Autodesk Inventor part; units mm, degrees
(part 3 of 3)
sketch "Sketch5" plane through (203.2, 0, 0) normal (0, 0, -1) x (-1, 0, 0)
  line L0 (0, 0) -> (203.2, 0) projected
  line L1 (0, 0) -> (0, -25.4) projected
  line L2 (203.2, -25.4) -> (0, -25.4) projected
  line L3 (203.2, 0) -> (203.2, -25.4) projected
  line L4 (12.7, -4.254) -> (190.5, -4.254) construction
  line L5 (190.5, -4.254) -> (190.5, -21.146) construction
  line L6 (190.5, -21.146) -> (12.7, -21.146) construction
  line L7 (12.7, -21.146) -> (12.7, -4.254) construction
  line L8 (18.2258, -17.272) -> (18.2258, -9.2099)
  line L9 (18.2258, -9.2099) -> (15.1581, -9.2099)
  line L10 (15.1581, -9.2099) -> (15.1581, -8.128)
  line L11 (15.1581, -8.128) -> (22.5088, -8.128)
  line L12 (22.5088, -8.128) -> (22.5088, -9.2099)
  line L13 (22.5088, -9.2099) -> (19.4411, -9.2099)
  line L14 (19.4411, -9.2099) -> (19.4411, -17.272)
  line L15 (19.4411, -17.272) -> (18.2258, -17.272)
  line L16 (30.5117, -17.272) -> (28.9334, -17.272)
  line L17 (28.9334, -17.272) -> (26.0434, -13.6337)
  line L18 (26.0434, -13.6337) -> (24.6504, -13.6337)
  line L19 (24.6504, -13.6337) -> (24.6504, -17.272)
  line L20 (24.6504, -17.272) -> (23.4351, -17.272)
  line L21 (23.4351, -17.272) -> (23.4351, -8.128)
  line L22 (23.4351, -8.128) -> (25.7915, -8.128)
  spline S0 degree 2 poles (25.7915, -8.128) (26.577, -8.128) (27.6366, -8.2984) (28.1183, -8.6097) knots 0 0 0 1 2 2 2
  spline S1 degree 2 poles (28.1183, -8.6097) (28.5999, -8.9209) (29.1557, -9.8916) (29.1557, -10.6104) knots 0 0 0 1 2 2 2
  spline S2 degree 2 poles (29.1557, -10.6104) (29.1557, -11.6107) (28.1331, -12.9668) (27.2587, -13.2928) knots 0 0 0 1 2 2 2
  line L23 (27.2587, -13.2928) -> (30.5117, -17.272)
  spline S3 degree 2 poles (27.8885, -10.7067) (27.8885, -10.3066) (27.607, -9.6915) (27.3106, -9.4914) knots 0 0 0 1 2 2 2
  spline S4 degree 2 poles (27.3106, -9.4914) (27.0512, -9.321) (26.3621, -9.1802) (25.8582, -9.1802) knots 0 0 0 1 2 2 2
  line L24 (25.8582, -9.1802) -> (24.6504, -9.1802)
  line L25 (24.6504, -9.1802) -> (24.6504, -12.6185)
  line L26 (24.6504, -12.6185) -> (25.7174, -12.6185)
  spline S5 degree 2 poles (25.7174, -12.6185) (26.2435, -12.6185) (27.0808, -12.4332) (27.3698, -12.1442) knots 0 0 0 1 2 2 2
  spline S6 degree 2 poles (27.3698, -12.1442) (27.6366, -11.8923) (27.8885, -11.1809) (27.8885, -10.7067) knots 0 0 0 1 2 2 2
  line L27 (31.2379, -17.272) -> (31.2379, -8.128)
  line L28 (31.2379, -8.128) -> (36.9584, -8.128)
  line L29 (36.9584, -8.128) -> (36.9584, -9.2099)
  line L30 (36.9584, -9.2099) -> (32.4531, -9.2099)
  line L31 (32.4531, -9.2099) -> (32.4531, -11.7145)
  line L32 (32.4531, -11.7145) -> (36.6546, -11.7145)
  line L33 (36.6546, -11.7145) -> (36.6546, -12.7963)
  line L34 (36.6546, -12.7963) -> (32.4531, -12.7963)
  line L35 (32.4531, -12.7963) -> (32.4531, -16.1901)
  line L36 (32.4531, -16.1901) -> (36.9584, -16.1901)
  line L37 (36.9584, -16.1901) -> (36.9584, -17.272)
  line L38 (36.9584, -17.272) -> (31.2379, -17.272)
  spline S7 degree 2 poles (44.4945, -14.4636) (44.4945, -15.1453) (43.9758, -16.1901) (43.546, -16.531) knots 0 0 0 1 2 2 2
  spline S8 degree 2 poles (43.546, -16.531) (43.0273, -16.9311) (41.8491, -17.272) (40.9154, -17.272) knots 0 0 0 1 2 2 2
  line L39 (40.9154, -17.272) -> (38.2923, -17.272)
  line L40 (38.2923, -17.272) -> (38.2923, -8.128)
  line L41 (38.2923, -8.128) -> (40.7153, -8.128)
  spline S9 degree 2 poles (40.7153, -8.128) (41.6935, -8.128) (42.6716, -8.254) (43.1162, -8.4985) knots 0 0 0 1 2 2 2
  spline S10 degree 2 poles (43.1162, -8.4985) (43.6127, -8.7579) (44.0647, -9.61) (44.0647, -10.188) knots 0 0 0 1 2 2 2
  spline S11 degree 2 poles (44.0647, -10.188) (44.0647, -10.8327) (43.383, -11.8553) (42.7827, -12.1442) knots 0 0 0 1 2 2 2
  line L42 (42.7827, -12.1442) -> (42.7827, -12.1887)
  spline S12 degree 2 poles (42.7827, -12.1887) (43.5978, -12.411) (44.4945, -13.5892) (44.4945, -14.4636) knots 0 0 0 1 2 2 2
  spline S13 degree 2 poles (43.2273, -14.5155) (43.2273, -13.9968) (42.9309, -13.3299) (42.4863, -13.0927) knots 0 0 0 1 2 2 2
  spline S14 degree 2 poles (42.4863, -13.0927) (42.1973, -12.9445) (41.5156, -12.8556) (40.8858, -12.8556) knots 0 0 0 1 2 2 2
  line L43 (40.8858, -12.8556) -> (39.5075, -12.8556)
  line L44 (39.5075, -12.8556) -> (39.5075, -16.2346)
  line L45 (39.5075, -16.2346) -> (40.493, -16.2346)
  spline S15 degree 2 poles (40.493, -16.2346) (41.2933, -16.2346) (42.2122, -16.0864) (42.5679, -15.8493) knots 0 0 0 1 2 2 2
  spline S16 degree 2 poles (42.5679, -15.8493) (42.9087, -15.6047) (43.2273, -14.9971) (43.2273, -14.5155) knots 0 0 0 1 2 2 2
  spline S17 degree 2 poles (42.7976, -10.3584) (42.7976, -10.0324) (42.5753, -9.5433) (42.3307, -9.4025) knots 0 0 0 1 2 2 2
  spline S18 degree 2 poles (42.3307, -9.4025) (42.0343, -9.2395) (41.3156, -9.1654) (40.6709, -9.1654) knots 0 0 0 1 2 2 2
  line L46 (40.6709, -9.1654) -> (39.5075, -9.1654)
  line L47 (39.5075, -9.1654) -> (39.5075, -11.8404)
  line L48 (39.5075, -11.8404) -> (40.8858, -11.8404)
  spline S19 degree 2 poles (40.8858, -11.8404) (41.4563, -11.8404) (41.9973, -11.7219) (42.2863, -11.5366) knots 0 0 0 1 2 2 2
  spline S20 degree 2 poles (42.2863, -11.5366) (42.5679, -11.3588) (42.7976, -10.7882) (42.7976, -10.3584) knots 0 0 0 1 2 2 2
  line L49 (51.0005, -17.272) -> (45.7023, -17.272)
  line L50 (45.7023, -17.272) -> (45.7023, -8.128)
  line L51 (45.7023, -8.128) -> (46.9175, -8.128)
  line L52 (46.9175, -8.128) -> (46.9175, -16.1901)
  line L53 (46.9175, -16.1901) -> (51.0005, -16.1901)
  line L54 (51.0005, -16.1901) -> (51.0005, -17.272)
  line L55 (51.9564, -17.272) -> (51.9564, -8.128)
  line L56 (51.9564, -8.128) -> (57.6769, -8.128)
  line L57 (57.6769, -8.128) -> (57.6769, -9.2099)
  line L58 (57.6769, -9.2099) -> (53.1716, -9.2099)
  line L59 (53.1716, -9.2099) -> (53.1716, -11.7145)
  line L60 (53.1716, -11.7145) -> (57.3731, -11.7145)
  line L61 (57.3731, -11.7145) -> (57.3731, -12.7963)
  line L62 (57.3731, -12.7963) -> (53.1716, -12.7963)
  line L63 (53.1716, -12.7963) -> (53.1716, -16.1901)
  line L64 (53.1716, -16.1901) -> (57.6769, -16.1901)
  line L65 (57.6769, -16.1901) -> (57.6769, -17.272)
  line L66 (57.6769, -17.272) -> (51.9564, -17.272)
  line L67 (68.4067, -9.2099) -> (64.1533, -9.2099)
  line L68 (64.1533, -9.2099) -> (64.1533, -11.7886)
  line L69 (64.1533, -11.7886) -> (68.2288, -11.7886)
  line L70 (68.2288, -11.7886) -> (68.2288, -12.8704)
  line L71 (68.2288, -12.8704) -> (64.1533, -12.8704)
  line L72 (64.1533, -12.8704) -> (64.1533, -17.272)
  line L73 (64.1533, -17.272) -> (62.9381, -17.272)
  line L74 (62.9381, -17.272) -> (62.9381, -8.128)
  line L75 (62.9381, -8.128) -> (68.4067, -8.128)
  line L76 (68.4067, -8.128) -> (68.4067, -9.2099)
  spline S21 degree 2 poles (75.9649, -9.1728) (76.4836, -9.7804) (77.0616, -11.5589) (77.0616, -12.7) knots 0 0 0 1 2 2 2
  spline S22 degree 2 poles (77.0616, -12.7) (77.0616, -13.8115) (76.4985, -15.6121) (75.9649, -16.2198) knots 0 0 0 1 2 2 2
  spline S23 degree 2 poles (75.9649, -16.2198) (75.4018, -16.857) (73.9124, -17.4647) (73.0157, -17.4647) knots 0 0 0 1 2 2 2
  spline S24 degree 2 poles (73.0157, -17.4647) (72.0895, -17.4647) (70.6075, -16.8348) (70.0665, -16.2198) knots 0 0 0 1 2 2 2
  spline S25 degree 2 poles (70.0665, -16.2198) (69.5404, -15.6121) (68.9773, -13.8263) (68.9773, -12.7) knots 0 0 0 1 2 2 2
  spline S26 degree 2 poles (68.9773, -12.7) (68.9773, -11.5514) (69.5478, -9.8027) (70.074, -9.1728) knots 0 0 0 1 2 2 2
  spline S27 degree 2 poles (70.074, -9.1728) (70.6075, -8.5652) (72.0969, -7.9353) (73.0157, -7.9353) knots 0 0 0 1 2 2 2
  spline S28 degree 2 poles (73.0157, -7.9353) (73.9494, -7.9353) (75.4462, -8.5874) (75.9649, -9.1728) knots 0 0 0 1 2 2 2
  spline S29 degree 2 poles (75.7945, -12.7) (75.7945, -11.796) (75.4018, -10.3955) (75.0461, -9.9361) knots 0 0 0 1 2 2 2
  spline S30 degree 2 poles (75.0461, -9.9361) (74.683, -9.4618) (73.6604, -8.9876) (73.0231, -8.9876) knots 0 0 0 1 2 2 2
  spline S31 degree 2 poles (73.0231, -8.9876) (72.3637, -8.9876) (71.3707, -9.447) (70.9928, -9.9361) knots 0 0 0 1 2 2 2
  spline S32 degree 2 poles (70.9928, -9.9361) (70.6297, -10.4029) (70.2444, -11.8108) (70.2444, -12.7) knots 0 0 0 1 2 2 2
  spline S33 degree 2 poles (70.2444, -12.7) (70.2444, -14.5006) (71.756, -16.4124) (73.0231, -16.4124) knots 0 0 0 1 2 2 2
  spline S34 degree 2 poles (73.0231, -16.4124) (74.2903, -16.4124) (75.7945, -14.5006) (75.7945, -12.7) knots 0 0 0 1 2 2 2
  spline S35 degree 2 poles (81.5892, -17.4647) (80.7815, -17.4647) (79.581, -17.0423) (79.1587, -16.6199) knots 0 0 0 1 2 2 2
  spline S36 degree 2 poles (79.1587, -16.6199) (78.677, -16.1457) (78.2843, -14.8119) (78.2843, -13.8337) knots 0 0 0 1 2 2 2
  line L77 (78.2843, -13.8337) -> (78.2843, -8.128)
  line L78 (78.2843, -8.128) -> (79.4995, -8.128)
  line L79 (79.4995, -8.128) -> (79.4995, -13.8337)
  spline S37 degree 2 poles (79.4995, -13.8337) (79.4995, -14.471) (79.6626, -15.3306) (79.8923, -15.6788) knots 0 0 0 1 2 2 2
  spline S38 degree 2 poles (79.8923, -15.6788) (80.1368, -16.0493) (80.9815, -16.4273) (81.5892, -16.4273) knots 0 0 0 1 2 2 2
  spline S39 degree 2 poles (81.5892, -16.4273) (82.1597, -16.4273) (83.0489, -16.0493) (83.2935, -15.6788) knots 0 0 0 1 2 2 2
  spline S40 degree 2 poles (83.2935, -15.6788) (83.5232, -15.3306) (83.6862, -14.4784) (83.6862, -13.8634) knots 0 0 0 1 2 2 2
  line L80 (83.6862, -13.8634) -> (83.6862, -8.128)
  line L81 (83.6862, -8.128) -> (84.9015, -8.128)
  line L82 (84.9015, -8.128) -> (84.9015, -13.8337)
  spline S41 degree 2 poles (84.9015, -13.8337) (84.9015, -14.7896) (84.5161, -16.1531) (84.0271, -16.6199) knots 0 0 0 1 2 2 2
  spline S42 degree 2 poles (84.0271, -16.6199) (83.5899, -17.0497) (82.4339, -17.4647) (81.5892, -17.4647) knots 0 0 0 1 2 2 2
  line L83 (93.7194, -17.272) -> (92.1411, -17.272)
  line L84 (92.1411, -17.272) -> (89.2512, -13.6337)
  line L85 (89.2512, -13.6337) -> (87.8581, -13.6337)
  line L86 (87.8581, -13.6337) -> (87.8581, -17.272)
  line L87 (87.8581, -17.272) -> (86.6428, -17.272)
  line L88 (86.6428, -17.272) -> (86.6428, -8.128)
  line L89 (86.6428, -8.128) -> (88.9992, -8.128)
  spline S43 degree 2 poles (88.9992, -8.128) (89.7847, -8.128) (90.8443, -8.2984) (91.326, -8.6097) knots 0 0 0 1 2 2 2
  spline S44 degree 2 poles (91.326, -8.6097) (91.8076, -8.9209) (92.3634, -9.8916) (92.3634, -10.6104) knots 0 0 0 1 2 2 2
  spline S45 degree 2 poles (92.3634, -10.6104) (92.3634, -11.6107) (91.3408, -12.9668) (90.4664, -13.2928) knots 0 0 0 1 2 2 2
  line L90 (90.4664, -13.2928) -> (93.7194, -17.272)
  spline S46 degree 2 poles (91.0963, -10.7067) (91.0963, -10.3066) (90.8147, -9.6915) (90.5183, -9.4914) knots 0 0 0 1 2 2 2
  spline S47 degree 2 poles (90.5183, -9.4914) (90.2589, -9.321) (89.5698, -9.1802) (89.0659, -9.1802) knots 0 0 0 1 2 2 2
  line L91 (89.0659, -9.1802) -> (87.8581, -9.1802)
  line L92 (87.8581, -9.1802) -> (87.8581, -12.6185)
  line L93 (87.8581, -12.6185) -> (88.9251, -12.6185)
  spline S48 degree 2 poles (88.9251, -12.6185) (89.4512, -12.6185) (90.2886, -12.4332) (90.5776, -12.1442) knots 0 0 0 1 2 2 2
  spline S49 degree 2 poles (90.5776, -12.1442) (90.8443, -11.8923) (91.0963, -11.1809) (91.0963, -10.7067) knots 0 0 0 1 2 2 2
  line L94 (97.6319, -17.272) -> (94.0899, -17.272)
  line L95 (94.0899, -17.272) -> (94.0899, -16.3383)
  line L96 (94.0899, -16.3383) -> (95.2533, -16.3383)
  line L97 (95.2533, -16.3383) -> (95.2533, -9.0617)
  line L98 (95.2533, -9.0617) -> (94.0899, -9.0617)
  line L99 (94.0899, -9.0617) -> (94.0899, -8.128)
  line L100 (94.0899, -8.128) -> (97.6319, -8.128)
  line L101 (97.6319, -8.128) -> (97.6319, -9.0617)
  line L102 (97.6319, -9.0617) -> (96.4685, -9.0617)
  line L103 (96.4685, -9.0617) -> (96.4685, -16.3383)
  line L104 (96.4685, -16.3383) -> (97.6319, -16.3383)
  line L105 (97.6319, -16.3383) -> (97.6319, -17.272)
  line L106 (99.1362, -17.272) -> (99.1362, -8.128)
  line L107 (99.1362, -8.128) -> (104.8567, -8.128)
  line L108 (104.8567, -8.128) -> (104.8567, -9.2099)
  line L109 (104.8567, -9.2099) -> (100.3514, -9.2099)
  line L110 (100.3514, -9.2099) -> (100.3514, -11.7145)
  line L111 (100.3514, -11.7145) -> (104.5529, -11.7145)
  line L112 (104.5529, -11.7145) -> (104.5529, -12.7963)
  line L113 (104.5529, -12.7963) -> (100.3514, -12.7963)
  line L114 (100.3514, -12.7963) -> (100.3514, -16.1901)
  line L115 (100.3514, -16.1901) -> (104.8567, -16.1901)
  line L116 (104.8567, -16.1901) -> (104.8567, -17.272)
  line L117 (104.8567, -17.272) -> (99.1362, -17.272)
  line L118 (113.2671, -17.272) -> (111.6888, -17.272)
  line L119 (111.6888, -17.272) -> (108.7989, -13.6337)
  line L120 (108.7989, -13.6337) -> (107.4058, -13.6337)
  line L121 (107.4058, -13.6337) -> (107.4058, -17.272)
  line L122 (107.4058, -17.272) -> (106.1905, -17.272)
  line L123 (106.1905, -17.272) -> (106.1905, -8.128)
  line L124 (106.1905, -8.128) -> (108.5469, -8.128)
  spline S50 degree 2 poles (108.5469, -8.128) (109.3324, -8.128) (110.392, -8.2984) (110.8737, -8.6097) knots 0 0 0 1 2 2 2
  spline S51 degree 2 poles (110.8737, -8.6097) (111.3553, -8.9209) (111.9111, -9.8916) (111.9111, -10.6104) knots 0 0 0 1 2 2 2
  spline S52 degree 2 poles (111.9111, -10.6104) (111.9111, -11.6107) (110.8885, -12.9668) (110.0141, -13.2928) knots 0 0 0 1 2 2 2
  line L125 (110.0141, -13.2928) -> (113.2671, -17.272)
  spline S53 degree 2 poles (110.644, -10.7067) (110.644, -10.3066) (110.3624, -9.6915) (110.066, -9.4914) knots 0 0 0 1 2 2 2
  spline S54 degree 2 poles (110.066, -9.4914) (109.8066, -9.321) (109.1175, -9.1802) (108.6136, -9.1802) knots 0 0 0 1 2 2 2
  line L126 (108.6136, -9.1802) -> (107.4058, -9.1802)
  line L127 (107.4058, -9.1802) -> (107.4058, -12.6185)
  line L128 (107.4058, -12.6185) -> (108.4728, -12.6185)
  spline S55 degree 2 poles (108.4728, -12.6185) (108.9989, -12.6185) (109.8363, -12.4332) (110.1253, -12.1442) knots 0 0 0 1 2 2 2
  spline S56 degree 2 poles (110.1253, -12.1442) (110.392, -11.8923) (110.644, -11.1809) (110.644, -10.7067) knots 0 0 0 1 2 2 2
  line L129 (120.0547, -17.272) -> (120.0547, -9.2099)
  line L130 (120.0547, -9.2099) -> (116.987, -9.2099)
  line L131 (116.987, -9.2099) -> (116.987, -8.128)
  line L132 (116.987, -8.128) -> (124.3377, -8.128)
  line L133 (124.3377, -8.128) -> (124.3377, -9.2099)
  line L134 (124.3377, -9.2099) -> (121.27, -9.2099)
  line L135 (121.27, -9.2099) -> (121.27, -17.272)
  line L136 (121.27, -17.272) -> (120.0547, -17.272)
  line L137 (132.3406, -17.272) -> (130.7622, -17.272)
  line L138 (130.7622, -17.272) -> (127.8723, -13.6337)
  line L139 (127.8723, -13.6337) -> (126.4792, -13.6337)
  line L140 (126.4792, -13.6337) -> (126.4792, -17.272)
  line L141 (126.4792, -17.272) -> (125.264, -17.272)
  line L142 (125.264, -17.272) -> (125.264, -8.128)
  line L143 (125.264, -8.128) -> (127.6204, -8.128)
  spline S57 degree 2 poles (127.6204, -8.128) (128.4059, -8.128) (129.4655, -8.2984) (129.9471, -8.6097) knots 0 0 0 1 2 2 2
  spline S58 degree 2 poles (129.9471, -8.6097) (130.4288, -8.9209) (130.9845, -9.8916) (130.9845, -10.6104) knots 0 0 0 1 2 2 2
  spline S59 degree 2 poles (130.9845, -10.6104) (130.9845, -11.6107) (129.962, -12.9668) (129.0876, -13.2928) knots 0 0 0 1 2 2 2
  line L144 (129.0876, -13.2928) -> (132.3406, -17.272)
  spline S60 degree 2 poles (129.7174, -10.7067) (129.7174, -10.3066) (129.4358, -9.6915) (129.1394, -9.4914) knots 0 0 0 1 2 2 2
  spline S61 degree 2 poles (129.1394, -9.4914) (128.8801, -9.321) (128.191, -9.1802) (127.6871, -9.1802) knots 0 0 0 1 2 2 2
  line L145 (127.6871, -9.1802) -> (126.4792, -9.1802)
  line L146 (126.4792, -9.1802) -> (126.4792, -12.6185)
  line L147 (126.4792, -12.6185) -> (127.5463, -12.6185)
  spline S62 degree 2 poles (127.5463, -12.6185) (128.0724, -12.6185) (128.9097, -12.4332) (129.1987, -12.1442) knots 0 0 0 1 2 2 2
  spline S63 degree 2 poles (129.1987, -12.1442) (129.4655, -11.8923) (129.7174, -11.1809) (129.7174, -10.7067) knots 0 0 0 1 2 2 2
  line L148 (132.0812, -17.272) -> (135.1638, -8.128)
  line L149 (135.1638, -8.128) -> (136.6606, -8.128)
  line L150 (136.6606, -8.128) -> (139.7432, -17.272)
  line L151 (139.7432, -17.272) -> (138.4613, -17.272)
  line L152 (138.4613, -17.272) -> (137.6314, -14.7155)
  line L153 (137.6314, -14.7155) -> (134.1412, -14.7155)
  line L154 (134.1412, -14.7155) -> (133.3113, -17.272)
  line L155 (133.3113, -17.272) -> (132.0812, -17.272)
  line L156 (137.2979, -13.6781) -> (135.8826, -9.3729)
  line L157 (135.8826, -9.3729) -> (134.4747, -13.6781)
  line L158 (134.4747, -13.6781) -> (137.2979, -13.6781)
  line L159 (147.1533, -17.272) -> (145.7898, -17.272)
  line L160 (145.7898, -17.272) -> (141.7439, -9.3877)
  line L161 (141.7439, -9.3877) -> (141.7439, -17.272)
  line L162 (141.7439, -17.272) -> (140.6102, -17.272)
  line L163 (140.6102, -17.272) -> (140.6102, -8.128)
  line L164 (140.6102, -8.128) -> (142.3367, -8.128)
  line L165 (142.3367, -8.128) -> (146.0195, -15.3676)
  line L166 (146.0195, -15.3676) -> (146.0195, -8.128)
  line L167 (146.0195, -8.128) -> (147.1533, -8.128)
  line L168 (147.1533, -8.128) -> (147.1533, -17.272)
  spline S64 degree 2 poles (151.5548, -17.435) (150.5619, -17.435) (149.1688, -17.0201) (148.5538, -16.7237) knots 0 0 0 1 2 2 2
  line L169 (148.5538, -16.7237) -> (148.5538, -15.1972)
  line L170 (148.5538, -15.1972) -> (148.6427, -15.1972)
  spline S65 degree 2 poles (148.6427, -15.1972) (149.2429, -15.7604) (150.762, -16.3828) (151.4659, -16.3828) knots 0 0 0 1 2 2 2
  spline S66 degree 2 poles (151.4659, -16.3828) (152.4737, -16.3828) (153.5037, -15.5455) (153.5037, -14.8563) knots 0 0 0 1 2 2 2
  spline S67 degree 2 poles (153.5037, -14.8563) (153.5037, -14.308) (152.9628, -13.6263) (152.3774, -13.4558) knots 0 0 0 1 2 2 2
  spline S68 degree 2 poles (152.3774, -13.4558) (151.955, -13.3373) (151.251, -13.1742) (150.7249, -13.0409) knots 0 0 0 1 2 2 2
  spline S69 degree 2 poles (150.7249, -13.0409) (150.2507, -12.9149) (149.5023, -12.537) (149.2133, -12.2332) knots 0 0 0 1 2 2 2
  spline S70 degree 2 poles (149.2133, -12.2332) (148.9317, -11.9294) (148.6205, -11.1142) (148.6205, -10.5807) knots 0 0 0 1 2 2 2
  spline S71 degree 2 poles (148.6205, -10.5807) (148.6205, -9.4692) (150.3544, -7.965) (151.6956, -7.965) knots 0 0 0 1 2 2 2
  spline S72 degree 2 poles (151.6956, -7.965) (152.4663, -7.965) (153.8297, -8.2688) (154.4151, -8.5578) knots 0 0 0 1 2 2 2
  line L171 (154.4151, -8.5578) -> (154.4151, -10.0102)
  line L172 (154.4151, -10.0102) -> (154.3262, -10.0102)
  spline S73 degree 2 poles (154.3262, -10.0102) (153.889, -9.61) (152.5256, -9.0172) (151.7771, -9.0172) knots 0 0 0 1 2 2 2
  spline S74 degree 2 poles (151.7771, -9.0172) (150.9324, -9.0172) (149.8876, -9.8101) (149.8876, -10.4548) knots 0 0 0 1 2 2 2
  spline S75 degree 2 poles (149.8876, -10.4548) (149.8876, -11.0327) (150.5026, -11.7219) (151.0806, -11.8775) knots 0 0 0 1 2 2 2
  spline S76 degree 2 poles (151.0806, -11.8775) (151.4659, -11.9812) (152.5848, -12.248) (152.9553, -12.3591) knots 0 0 0 1 2 2 2
  spline S77 degree 2 poles (152.9553, -12.3591) (153.8964, -12.6481) (154.7708, -13.8115) (154.7708, -14.6637) knots 0 0 0 1 2 2 2
  spline S78 degree 2 poles (154.7708, -14.6637) (154.7708, -15.2046) (154.3336, -16.242) (153.9409, -16.6051) knots 0 0 0 1 2 2 2
  spline S79 degree 2 poles (153.9409, -16.6051) (153.5037, -17.0052) (152.3922, -17.435) (151.5548, -17.435) knots 0 0 0 1 2 2 2
  line L173 (161.4769, -9.2099) -> (157.2235, -9.2099)
  line L174 (157.2235, -9.2099) -> (157.2235, -11.7886)
  line L175 (157.2235, -11.7886) -> (161.2991, -11.7886)
  line L176 (161.2991, -11.7886) -> (161.2991, -12.8704)
  line L177 (161.2991, -12.8704) -> (157.2235, -12.8704)
  line L178 (157.2235, -12.8704) -> (157.2235, -17.272)
  line L179 (157.2235, -17.272) -> (156.0083, -17.272)
  line L180 (156.0083, -17.272) -> (156.0083, -8.128)
  line L181 (156.0083, -8.128) -> (161.4769, -8.128)
  line L182 (161.4769, -8.128) -> (161.4769, -9.2099)
  spline S80 degree 2 poles (169.0351, -9.1728) (169.5539, -9.7804) (170.1318, -11.5589) (170.1318, -12.7) knots 0 0 0 1 2 2 2
  spline S81 degree 2 poles (170.1318, -12.7) (170.1318, -13.8115) (169.5687, -15.6121) (169.0351, -16.2198) knots 0 0 0 1 2 2 2
  spline S82 degree 2 poles (169.0351, -16.2198) (168.472, -16.857) (166.9826, -17.4647) (166.0859, -17.4647) knots 0 0 0 1 2 2 2
  spline S83 degree 2 poles (166.0859, -17.4647) (165.1597, -17.4647) (163.6777, -16.8348) (163.1367, -16.2198) knots 0 0 0 1 2 2 2
  spline S84 degree 2 poles (163.1367, -16.2198) (162.6106, -15.6121) (162.0475, -13.8263) (162.0475, -12.7) knots 0 0 0 1 2 2 2
  spline S85 degree 2 poles (162.0475, -12.7) (162.0475, -11.5514) (162.618, -9.8027) (163.1442, -9.1728) knots 0 0 0 1 2 2 2
  spline S86 degree 2 poles (163.1442, -9.1728) (163.6777, -8.5652) (165.1671, -7.9353) (166.0859, -7.9353) knots 0 0 0 1 2 2 2
  spline S87 degree 2 poles (166.0859, -7.9353) (167.0196, -7.9353) (168.5164, -8.5874) (169.0351, -9.1728) knots 0 0 0 1 2 2 2
  spline S88 degree 2 poles (168.8647, -12.7) (168.8647, -11.796) (168.472, -10.3955) (168.1163, -9.9361) knots 0 0 0 1 2 2 2
  spline S89 degree 2 poles (168.1163, -9.9361) (167.7532, -9.4618) (166.7306, -8.9876) (166.0934, -8.9876) knots 0 0 0 1 2 2 2
  spline S90 degree 2 poles (166.0934, -8.9876) (165.4339, -8.9876) (164.4409, -9.447) (164.063, -9.9361) knots 0 0 0 1 2 2 2
  spline S91 degree 2 poles (164.063, -9.9361) (163.6999, -10.4029) (163.3146, -11.8108) (163.3146, -12.7) knots 0 0 0 1 2 2 2
  spline S92 degree 2 poles (163.3146, -12.7) (163.3146, -14.5006) (164.8262, -16.4124) (166.0934, -16.4124) knots 0 0 0 1 2 2 2
  spline S93 degree 2 poles (166.0934, -16.4124) (167.3605, -16.4124) (168.8647, -14.5006) (168.8647, -12.7) knots 0 0 0 1 2 2 2
  line L183 (178.5422, -17.272) -> (176.9639, -17.272)
  line L184 (176.9639, -17.272) -> (174.074, -13.6337)
  line L185 (174.074, -13.6337) -> (172.6809, -13.6337)
  line L186 (172.6809, -13.6337) -> (172.6809, -17.272)
  line L187 (172.6809, -17.272) -> (171.4656, -17.272)
  line L188 (171.4656, -17.272) -> (171.4656, -8.128)
  line L189 (171.4656, -8.128) -> (173.822, -8.128)
  spline S94 degree 2 poles (173.822, -8.128) (174.6075, -8.128) (175.6671, -8.2984) (176.1488, -8.6097) knots 0 0 0 1 2 2 2
  spline S95 degree 2 poles (176.1488, -8.6097) (176.6304, -8.9209) (177.1862, -9.8916) (177.1862, -10.6104) knots 0 0 0 1 2 2 2
  spline S96 degree 2 poles (177.1862, -10.6104) (177.1862, -11.6107) (176.1636, -12.9668) (175.2892, -13.2928) knots 0 0 0 1 2 2 2
  line L190 (175.2892, -13.2928) -> (178.5422, -17.272)
  spline S97 degree 2 poles (175.9191, -10.7067) (175.9191, -10.3066) (175.6375, -9.6915) (175.3411, -9.4914) knots 0 0 0 1 2 2 2
  spline S98 degree 2 poles (175.3411, -9.4914) (175.0817, -9.321) (174.3926, -9.1802) (173.8887, -9.1802) knots 0 0 0 1 2 2 2
  line L191 (173.8887, -9.1802) -> (172.6809, -9.1802)
  line L192 (172.6809, -9.1802) -> (172.6809, -12.6185)
  line L193 (172.6809, -12.6185) -> (173.7479, -12.6185)
  spline S99 degree 2 poles (173.7479, -12.6185) (174.2741, -12.6185) (175.1114, -12.4332) (175.4004, -12.1442) knots 0 0 0 1 2 2 2
  spline S100 degree 2 poles (175.4004, -12.1442) (175.6671, -11.8923) (175.9191, -11.1809) (175.9191, -10.7067) knots 0 0 0 1 2 2 2
  line L194 (187.1083, -17.272) -> (185.893, -17.272)
  line L195 (185.893, -17.272) -> (185.893, -9.3951)
  line L196 (185.893, -9.3951) -> (183.507, -14.7526)
  line L197 (183.507, -14.7526) -> (182.766, -14.7526)
  line L198 (182.766, -14.7526) -> (180.4022, -9.3951)
  line L199 (180.4022, -9.3951) -> (180.4022, -17.272)
  line L200 (180.4022, -17.272) -> (179.2684, -17.272)
  line L201 (179.2684, -17.272) -> (179.2684, -8.128)
  line L202 (179.2684, -8.128) -> (180.9283, -8.128)
  line L203 (180.9283, -8.128) -> (183.2106, -13.2187)
  line L204 (183.2106, -13.2187) -> (185.4188, -8.128)
  line L205 (185.4188, -8.128) -> (187.1083, -8.128)
  line L206 (187.1083, -8.128) -> (187.1083, -17.272)
  dimension "d30" = 203.2
  dimension "d31" = 177.8
  dimension "d32" = 16.892
  dimension "d33" = 4.254
  dimension "d34" = 25.4
  dimension "d35" = 12.7
  constraints: 2 other
  measures "d30" distance of L0.start L0.end
  measures "d31" distance of L7.end L4.end
  measures "d32" distance of L7.start L7.end
  measures "d33" distance between parallel lines of L0 L4
  measures "d34" distance of L0.start L1.end
  measures "d35" distance between parallel lines of L1 L7
extrude "Extrusion5" cut sketch "Sketch5" against normal blind 5.08 contours L8 L9 L10 L11 L12 L13 L14 L15 | L16 L17 L18 L19 L20 L21 L22 S0 S1 S2 L23 | L27 L28 L29 L30 L31 L32 L33 L34 L35 L36 L37 L38 | S7 S8 L39 L40 L41 S9 S10 S11 L42 S12 | L49 L50 L51 L52 L53 L54 | L55 L56 L57 L58 L59 L60 L61 L62 L63 L64 L65 L66 | L67 L68 L69 L70 L71 L72 L73 L74 L75 L76 | S21 S22 S23 S24 S25 S26 S27 S28 | S35 S36 L77 L78 L79 S37 S38 S39 S40 L80 L81 L82 S41 S42 | L83 L84 L85 L86 L87 L88 L89 S43 S44 S45 L90 | L94 L95 L96 L97 L98 L99 L100 L101 L102 L103 L104 L105 | L106 L107 L108 L109 L110 L111 L112 L113 L114 L115 L116 L117 | L118 L119 L120 L121 L122 L123 L124 S50 S51 S52 L125 | L129 L130 L131 L132 L133 L134 L135 L136 | L137 L148 L144 | L144 L148 L149 L150 L151 L152 L153 L154 L155 | L137 L138 L139 L140 L141 L142 L143 S57 S58 S59 L144 L148 | L159 L160 L161 L162 L163 L164 L165 L166 L167 L168 | S64 L169 L170 S65 S66 S67 S68 S69 S70 S71 S72 L171 L172 S73 S74 S75 S76 S77 S78 S79 | L173 L174 L175 L176 L177 L178 L179 L180 L181 L182 | S80 S81 S82 S83 S84 S85 S86 S87 | L183 L184 L185 L186 L187 L188 L189 S94 S95 S96 L190 | L194 L195 L196 L197 L198 L199 L200 L201 L202 L203 L204 L205 L206
equation "\"d6\" = 0.5 * d3 - 0.5 * d5"
equation "\"d7\" = 0.5 * d2 - 0.5 * d4"
equation "\"d16\" = 0.5 * d15 - 0.5 * d11"
equation "\"d17\" = 0.5 * d15 - 0.5 * d13"
equation "\"d18\" = -0.333333 * d12 + 0.333333 * d14 - 0.333333 * d10"
equation "\"d19\" = d18"
equation "\"d26\" = 0.5 * d24 - 0.5 * d22"
equation "\"d27\" = 0.5 * d25 - 0.5 * d23"
equation "\"d33\" = 0.5 * d34 - 0.5 * d32"
equation "\"d35\" = 0.5 * d30 - 0.5 * d31"
body "Solid1"
